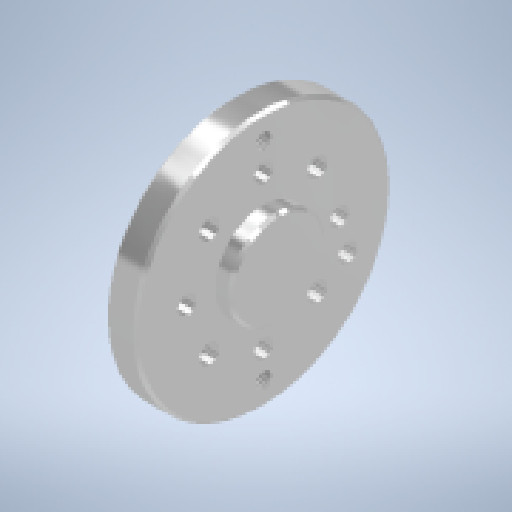
# Autodesk Inventor part: UR5 Gripper Interface plate
Saved by Autodesk Inventor 2025.1 (Build 291241000, 241)
## iProperties
Created: 2025-02-13
Part Number: UR5 Gripper Interface plate
Material: Aluminum 6061
Document SubType Name: Modeling
Designer: frede
Density: 2.7 g/cm^3
Appearance: Aluminum - Flat
Author: frede
Autodesk Inventor part; units mm, degrees
note: some values were not read from the file. Chosen so that the rebuilt part matches the saved one: direction of "Hole1"; direction of "Hole2"; direction of "Hole3"; direction of "Hole5".
ref_plane "YZ Plane" through (0, 0, 0) normal (1, 0, 0) x (0, 1, 0)
ref_plane "XZ Plane" through (0, 0, 0) normal (0, 1, 0) x (-1, 0, 0)
ref_plane "XY Plane" through (0, 0, 0) normal (0, 0, 1) x (1, 0, 0)
sketch "Sketch1" plane through (0, 0, 0) normal (0, 0, 1) x (1, 0, 0)
  line L0 (-15, 41) -> (-15, 16.75)
  line L1 (-14, 15.75) -> (-9, 15.75)
  line L2 (-9, 15.75) -> (-9, 0)
  line L3 (-9, 0) -> (0, 0)
  line L4 (0, 0) -> (0, 14.75)
  line L5 (-1, 15.75) -> (-5, 15.75)
  line L6 (-5, 15.75) -> (-5, 41)
  line L7 (-6, 42) -> (-14, 42)
  line L8 (-5, 41) -> (-6, 42)
  line L9 (-15, 41) -> (-14, 42)
  line L10 (-14, 15.75) -> (-15, 16.75)
  line L11 (-1, 15.75) -> (0, 14.75)
  point P0 (-15, 42)
  point P1 (-15, 15.75)
  point P2 (0, 15.75)
  point P3 (-5, 42)
  point P4 (0, 7.375)
  point P5 (-4.5, 0)
  point P6 (-10, 42)
  point P7 (-11.5, 15.75)
  dimension "d1" = 6
  dimension "d2" = 15.75
  dimension "d3" = 5
  dimension "d4" = 15
  dimension "d5" = 1
  dimension "d6" = 1
  dimension "d7" = 1
  dimension "d8" = 1
  dimension "d9" = 1
  dimension "d10" = 1
  dimension "d11" = 1
  dimension "d12" = 1
  dimension "d13" = 42
  dimension "d14" = 15.75
  constraints: 24 end point, 10 point on line, 5 perpendicular, 4 midpoint, 1 vertical
  measures "d1" distance of point (-15, 15.75) L1.end
  measures "d2" distance of L3.end point (0, 15.75)
  measures "d3" distance of point (0, 15.75) L5.end
  measures "d4" distance from line of point (0, 7.375) L0
  measures "d5" distance of L6.end point (-5, 42)
  measures "d6" distance of L7.start point (-5, 42)
  measures "d7" distance of L0.start point (-15, 42)
  measures "d8" distance of L7.end point (-15, 42)
  measures "d9" distance of L1.start point (-15, 15.75)
  measures "d10" distance of L0.end point (-15, 15.75)
  measures "d11" distance of L5.start point (0, 15.75)
  measures "d12" distance of L4.end point (0, 15.75)
  measures "d13" vertical distance of point (-4.5, 0) point (-10, 42)
  measures "d14" distance from line of L3 point (-11.5, 15.75)
revolve "Revolution1" add sketch "Sketch1" angle 360 about axis through (-9, 0, 0) along (1, 0, 0)
sketch "Sketch2" plane through (-5, 0, 0) normal (1, 0, 0) x (0, 0, -1)
  circle A0 centre (0, 0) radius 34
  circle A1 centre (0, 0) radius 30
  circle A2 centre (0, 0) radius 25
  circle A3 centre (0, 34) radius 2.5
  line L0 (0, 0) -> (42, 0)
  circle A4 centre (0, 0) radius 42 projected
  line L1 (27.7164, -11.4805) -> (0, 0)
  point P0 (0, -34)
  point P1 (0, 25)
  point P2 (0, -25)
  point P3 (-25, 0)
  point P4 (25, 0)
  point P5 (-17.6777, 17.6777)
  point P6 (17.6777, -17.6777)
  point P7 (-17.6777, -17.6777)
  point P8 (17.6777, 17.6777)
  dimension "d16" = 68
  dimension "d17" = 60
  dimension "d18" = 50
  dimension "d19" = 5
  dimension "d22" = 360
  dimension "d55" = -22.5
  constraints: 4 coincident, 4 end point, 4 point on circle, 2 centre point, 2 horizontal, 1 horizontal alignment, 1 vertical alignment, 9 other
  measures "d18" diameter of A2
  measures "d19" diameter of A3
  measures "d55" angle of L0 L1
hole "Hole1" at (-5, 34, 0) at (-5, -34, 0) direction (-1, 0, 0) diameter 4.917 depth 10 thread size "M6x1" class "6H" standard "ISO Metric profile"
hole "Hole2" at (-5, 25, 0) at (-5, 0, -25) at (-5, -25, 0) at (-5, 0, 25) direction (-1, 0, 0) diameter 6 end up to surface
hole "Hole3" at (-5, 17.6777, -17.6777) at (-5, -17.6777, -17.6777) at (-5, -17.6777, 17.6777) at (-5, 17.6777, 17.6777) direction (-1, 0, 0) diameter 6.4 end up to surface
hole "Hole5" at (-5, -11.4805, -27.7164) direction (-1, 0, 0) diameter 6 end up to surface
sketch "Sketch4" plane through (-15, 0, 0) normal (-1, 0, 0) x (0, 0, 1)
  circle A0 centre (-17.6777, 17.6777) radius 3.2 projected
  circle A1 centre (-17.6777, 17.6777) radius 5.5
  circle A2 centre (-17.6777, -17.6777) radius 5.5
  circle A3 centre (17.6777, -17.6777) radius 5.5
  circle A4 centre (17.6777, 17.6777) radius 5.5
  point P0 (0, 0)
  dimension "d63" = 11
  dimension "d66" = 360
  constraints: 4 centre point, 1 coincident, 9 other
  measures "d63" diameter of A1
extrude "Extrusion1" cut sketch "Sketch4" against normal blind 6.5 contours A0 | A1 | A2 | A3 | A4
equation "\"d6\" = d5"
equation "\"d7\" = d5"
equation "\"d8\" = d7"
equation "\"d9\" = d5"
equation "\"d10\" = d9"
equation "\"d11\" = d5"
equation "\"d12\" = d11"
body "Solid1"
